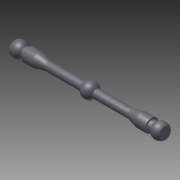
# Autodesk Inventor part: union
Saved by Autodesk Inventor 2012 (Build 160160000, 160)
## iProperties
Created: 2013-10-01
Part Number: union
Material: Default
Document SubType Name: Modeling
Designer: Nick
Density: 1 g/cm^3
Author: Nick
Autodesk Inventor part; units mm, degrees
ref_plane "YZ Plane" through (0, 0, 0) normal (1, 0, 0) x (0, 1, 0)
ref_plane "XZ Plane" through (0, 0, 0) normal (0, 1, 0) x (-1, 0, 0)
ref_plane "XY Plane" through (0, 0, 0) normal (0, 0, 1) x (1, 0, 0)
sketch "Sketch1" plane through (0, 0, 0) normal (0, 0, 1) x (1, 0, 0)
  line L0 (-3.1649, 3.1698) -> (44.3618, 3.1698) construction
  line L1 (4.6175, 4.4198) -> (17.1175, 4.4198) construction
  line L2 (-1.3825, 5.1698) -> (1.6175, 5.1698)
  line L3 (1.6175, 5.1698) -> (4.6175, 4.4198)
  line L4 (17.1175, 14.6605) -> (17.1175, -4.6585) construction
  line L5 (-1.3825, 5.1698) -> (-1.3825, 4.6698)
  line L6 (-1.3825, 4.6698) -> (-2.3825, 4.6698)
  circle A0 centre (-4.0584, 3.1698) radius 2.25 construction
  line L7 (-2.3825, 4.6698) -> (-5.3825, 4.6698) construction
  line L8 (-5.3825, 4.9889) -> (-5.3825, 3.1698)
  arc A1 (-2.3814, 4.6698) -> (-5.3825, 4.9889) centre (-4.0584, 3.1698) ccw
  line L9 (29.6175, 4.4198) -> (17.1175, 4.4198) construction
  line L10 (35.6175, 5.1698) -> (32.6175, 5.1698)
  line L11 (32.6175, 5.1698) -> (29.6175, 4.4198)
  line L12 (35.6175, 5.1698) -> (35.6175, 4.6698)
  line L13 (35.6175, 4.6698) -> (36.6175, 4.6698)
  circle A2 centre (38.2934, 3.1698) radius 2.25 construction
  line L14 (36.6175, 4.6698) -> (39.6175, 4.6698) construction
  line L15 (39.6175, 4.9889) -> (39.6175, 3.1698)
  arc A3 (39.6175, 4.9889) -> (36.6163, 4.6698) centre (38.2934, 3.1698) ccw
  line L16 (-5.3825, 3.1698) -> (39.6175, 3.1698)
  circle A4 centre (17.1175, 3.1698) radius 2.25 construction
  line L17 (4.6175, 4.4198) -> (15.2467, 4.4198)
  arc A5 (18.9883, 4.4198) -> (15.2467, 4.4198) centre (17.1175, 3.1698) ccw
  line L18 (18.9883, 4.4198) -> (29.6175, 4.4198)
  point P0 (37.3999, 3.1698)
  dimension "d1" = 1.25
  dimension "d2" = 12.5
  dimension "d3" = 2
  dimension "d4" = 3
  dimension "d5" = 3
  dimension "d6" = 1.5
  dimension "d7" = 1
  dimension "d8" = 4.5
  dimension "d9" = 3
  dimension "d11" = 4.5
  constraints: 38 end point, 12 point on circle, 12 symmetric about line, 6 centre point, 4 point on line, 3 collinear, 3 parallel, 3 perpendicular, 1 concentric, 1 horizontal, 1 midpoint, 2 other
  measures "d1" distance between parallel lines of L0 L1
  measures "d2" distance of L1.start L1.end
  measures "d3" distance between parallel lines of L0 L2
  measures "d4" distance of L2.start L2.end
  measures "d5" horizontal distance of L1.start L2.end
  measures "d6" vertical distance of L0.start L5.end
  measures "d7" distance of L5.end L6.end
  measures "d8" diameter of A0
  measures "d9" distance of L6.end L7.end
  measures "d11" diameter of A4
revolve "Revolution1" add sketch "Sketch1" angle 360 about axis through (-5.3825, 3.1698, 0) along (1, 0, 0)
equation "\"d11\" = d8"
body "Solid1"
